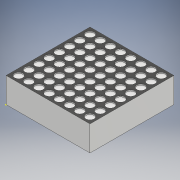
# Autodesk Inventor part: led2
Saved by Autodesk Inventor 2017 (Build 210142000, 142)
## iProperties
Part Number: led2
Material: Genérico
Document SubType Name: Modeling
Designer: Roberto
Density: 1 g/cm^3
Appearance: Valor por defecto
Author: Roberto
Autodesk Inventor part; units mm, degrees
ref_plane "YZ Plane" through (0, 0, 0) normal (1, 0, 0) x (0, 1, 0)
ref_plane "XZ Plane" through (0, 0, 0) normal (0, 1, 0) x (-1, 0, 0)
ref_plane "XY Plane" through (0, 0, 0) normal (0, 0, 1) x (1, 0, 0)
sketch "Boceto3" plane through (0, 0, 0) normal (0, 0, 1) x (1, 0, 0)
  line L0 (4, 0) -> (0, 0)
  line L1 (0, 0) -> (0, 4)
  line L2 (0, 4) -> (4, 4)
  line L3 (4, 4) -> (4, 0)
  constraints: 8 end point
extrude "Extrusión3" add sketch "Boceto3" along normal blind 1.15
sketch "Boceto4" plane through (0, 0, 1.15) normal (0, 0, 1) x (1, 0, 0)
  line L0 (4, 0) -> (0, 0)
  line L1 (0, 0) -> (0, 4)
  line L2 (0, 4) -> (4, 4)
  line L3 (4, 4) -> (4, 0)
  circle A0 centre (1.7575, 2.2425) radius 0.194
  circle A1 centre (1.2725, 2.2425) radius 0.194
  circle A2 centre (0.7875, 2.2425) radius 0.194
  circle A3 centre (0.3025, 2.2425) radius 0.194
  circle A4 centre (2.2425, 2.2425) radius 0.194
  circle A5 centre (2.7275, 2.2425) radius 0.194
  circle A6 centre (3.2125, 2.2425) radius 0.194
  circle A7 centre (3.6975, 2.2425) radius 0.194
  circle A8 centre (1.7575, 1.7575) radius 0.194
  circle A9 centre (1.2725, 1.7575) radius 0.194
  circle A10 centre (0.7875, 1.7575) radius 0.194
  circle A11 centre (0.3025, 1.7575) radius 0.194
  circle A12 centre (2.2425, 1.7575) radius 0.194
  circle A13 centre (2.7275, 1.7575) radius 0.194
  circle A14 centre (3.2125, 1.7575) radius 0.194
  circle A15 centre (3.6975, 1.7575) radius 0.194
  circle A16 centre (1.7575, 1.2725) radius 0.194
  circle A17 centre (1.2725, 1.2725) radius 0.194
  circle A18 centre (0.7875, 1.2725) radius 0.194
  circle A19 centre (0.3025, 1.2725) radius 0.194
  circle A20 centre (2.2425, 1.2725) radius 0.194
  circle A21 centre (2.7275, 1.2725) radius 0.194
  circle A22 centre (3.2125, 1.2725) radius 0.194
  circle A23 centre (3.6975, 1.2725) radius 0.194
  circle A24 centre (1.7575, 0.7875) radius 0.194
  circle A25 centre (1.2725, 0.7875) radius 0.194
  circle A26 centre (0.7875, 0.7875) radius 0.194
  circle A27 centre (0.3025, 0.7875) radius 0.194
  circle A28 centre (2.2425, 0.7875) radius 0.194
  circle A29 centre (2.7275, 0.7875) radius 0.194
  circle A30 centre (3.2125, 0.7875) radius 0.194
  circle A31 centre (3.6975, 0.7875) radius 0.194
  circle A32 centre (1.7575, 0.3025) radius 0.194
  circle A33 centre (1.2725, 0.3025) radius 0.194
  circle A34 centre (0.7875, 0.3025) radius 0.194
  circle A35 centre (0.3025, 0.3025) radius 0.194
  circle A36 centre (2.2425, 0.3025) radius 0.194
  circle A37 centre (2.7275, 0.3025) radius 0.194
  circle A38 centre (3.2125, 0.3025) radius 0.194
  circle A39 centre (3.6975, 0.3025) radius 0.194
  circle A40 centre (1.7575, 2.7275) radius 0.194
  circle A41 centre (1.2725, 2.7275) radius 0.194
  circle A42 centre (0.7875, 2.7275) radius 0.194
  circle A43 centre (0.3025, 2.7275) radius 0.194
  circle A44 centre (2.2425, 2.7275) radius 0.194
  circle A45 centre (2.7275, 2.7275) radius 0.194
  circle A46 centre (3.2125, 2.7275) radius 0.194
  circle A47 centre (3.6975, 2.7275) radius 0.194
  circle A48 centre (1.7575, 3.2125) radius 0.194
  circle A49 centre (1.2725, 3.2125) radius 0.194
  circle A50 centre (0.7875, 3.2125) radius 0.194
  circle A51 centre (0.3025, 3.2125) radius 0.194
  circle A52 centre (2.2425, 3.2125) radius 0.194
  circle A53 centre (2.7275, 3.2125) radius 0.194
  circle A54 centre (3.2125, 3.2125) radius 0.194
  circle A55 centre (3.6975, 3.2125) radius 0.194
  circle A56 centre (1.7575, 3.6975) radius 0.194
  circle A57 centre (1.2725, 3.6975) radius 0.194
  circle A58 centre (0.7875, 3.6975) radius 0.194
  circle A59 centre (0.3025, 3.6975) radius 0.194
  circle A60 centre (2.2425, 3.6975) radius 0.194
  circle A61 centre (2.7275, 3.6975) radius 0.194
  circle A62 centre (3.2125, 3.6975) radius 0.194
  circle A63 centre (3.6975, 3.6975) radius 0.194
  constraints: 64 centre point, 8 end point
extrude "Extrusión4" add sketch "Boceto4" along normal blind 0.05
sketch "Boceto5" plane through (0, 0, 0) normal (0, 0, -1) x (-1, 0, 0)
  point P0 (0, 0)
